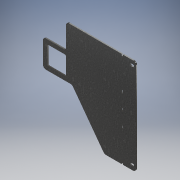
# Autodesk Inventor part: CAR SIDE PLATE II
Saved by Autodesk Inventor 2017 (Build 210142000, 142)
## iProperties
Part Number: CAR SIDE PLATE II
Material: Genérico
Document SubType Name: Modeling
Designer: Cristian
Density: 1 g/cm^3
Appearance: Valor por defecto
Author: Cristian
Autodesk Inventor part; units mm, degrees
ref_plane "YZ Plane" through (0, 0, 0) normal (1, 0, 0) x (0, 1, 0)
ref_plane "XZ Plane" through (0, 0, 0) normal (0, 1, 0) x (-1, 0, 0)
ref_plane "XY Plane" through (0, 0, 0) normal (0, 0, 1) x (1, 0, 0)
sketch "Boceto1" plane through (0, 0, 0) normal (0, 1, 0) x (-1, 0, 0)
  line L0 (0, 0) -> (288.925, 0)
  line L1 (288.925, 0) -> (288.925, -101.6)
  line L2 (288.925, -101.6) -> (384.175, -101.6)
  line L3 (384.175, -101.6) -> (384.175, -212.725)
  line L4 (0, 0) -> (0, -393.7)
  line L5 (0, -393.7) -> (130.175, -393.7)
  line L6 (384.175, -212.725) -> (263.525, -212.725)
  line L7 (263.525, -212.725) -> (130.175, -393.7)
  dimension "d0" = 288.925
  dimension "d1" = 101.6
  dimension "d2" = 95.25
  dimension "d3" = 111.125
  dimension "d4" = 393.7
  dimension "d50" = 130.175
  dimension "d51" = 133.35
  constraints: 16 end point, 3 horizontal, 2 perpendicular, 2 vertical
  measures "d0" distance of L0.start L0.end
  measures "d1" distance of L0.end L1.end
  measures "d2" distance of L1.end L2.end
  measures "d3" distance of L2.end L3.end
  measures "d4" distance of L0.start L4.end
  measures "d50" distance of L4.end L5.end
  measures "d51" horizontal distance of L5.end L6.end
extrude "Extrusión1" add sketch "Boceto1" along normal blind 5
fillet "Empalme1" radius 12.7 7 edges at (-384.175, 2.5, -101.6) (-288.925, 2.5, 0) (-384.175, 2.5, -212.725) (-263.525, 2.5, -212.725) (-130.175, 2.5, -393.7) (0, 2.5, -393.7) (0, 2.5, 0)
fillet "Empalme2" radius 6.35 1 edges at (-288.925, 2.5, -101.6)
sketch "Boceto2" plane through (0, 5, 0) normal (0, 1, 0) x (1, 0, 0)
  line L0 (-365.125, 119.0625) -> (-288.925, 119.0625)
  line L1 (-288.925, 119.0625) -> (-288.925, 195.2625)
  line L2 (-288.925, 195.2625) -> (-365.125, 195.2625)
  line L3 (-365.125, 195.2625) -> (-365.125, 119.0625)
  line L4 (-384.175, 200.025) -> (-384.175, 114.3) projected
  line L5 (-269.9424, 212.725) -> (-371.475, 212.725) projected
  line L6 (-371.475, 101.6) -> (-295.275, 101.6) projected
  line L7 (-276.225, 0) -> (-12.7, 0) projected
  line L8 (-59.5312, 0) -> (-53.975, 0)
  line L9 (-53.975, 0) -> (-53.975, 6.35)
  line L10 (-53.975, 6.35) -> (-59.5312, 6.35)
  line L11 (-59.5312, 6.35) -> (-59.5312, 0)
  line L12 (-12.7, 393.7) -> (-123.7576, 393.7) projected
  line L13 (0, 12.7) -> (0, 381) projected
  circle A0 centre (-15.875, 374.65) radius 5
  circle A1 centre (-15.875, 19.05) radius 5
  line L14 (-123.7576, 393.7) -> (-12.7, 393.7) projected
  line L15 (-59.5313, 393.7) -> (-53.975, 393.7)
  line L16 (-53.975, 393.7) -> (-53.975, 387.35)
  line L17 (-53.975, 387.35) -> (-59.5313, 387.35)
  line L18 (-59.5313, 387.35) -> (-59.5313, 393.7)
  line L19 (-59.5313, 127) -> (-53.975, 127)
  line L20 (-53.975, 127) -> (-53.975, 140.0969)
  line L21 (-53.975, 140.0969) -> (-59.5313, 140.0969)
  line L22 (-59.5313, 140.0969) -> (-59.5313, 127)
  line L23 (-59.5313, 190.5) -> (-53.975, 190.5)
  line L24 (-53.975, 190.5) -> (-53.975, 203.5969)
  line L25 (-53.975, 203.5969) -> (-59.5313, 203.5969)
  line L26 (-59.5313, 203.5969) -> (-59.5313, 190.5)
  line L27 (-59.5313, 254) -> (-53.975, 254)
  line L28 (-53.975, 254) -> (-53.975, 267.0969)
  line L29 (-53.975, 267.0969) -> (-59.5313, 267.0969)
  line L30 (-59.5313, 267.0969) -> (-59.5313, 254)
  circle A2 centre (-19.6062, 19.05) radius 5
  circle A3 centre (-12.1438, 19.05) radius 5
  line L31 (-19.6062, 19.05) -> (-15.875, 19.05)
  line L32 (-15.875, 19.05) -> (-12.1438, 19.05)
  line L33 (-19.6062, 14.05) -> (-12.1437, 14.05)
  line L34 (-19.6062, 24.05) -> (-12.1437, 24.05)
  circle A4 centre (-19.6063, 374.65) radius 5
  circle A5 centre (-12.1438, 374.65) radius 5
  line L35 (-19.6063, 374.65) -> (-15.875, 374.65)
  line L36 (-15.875, 374.65) -> (-12.1438, 374.65)
  line L37 (-19.6063, 369.65) -> (-12.1437, 369.65)
  line L38 (-19.6063, 379.65) -> (-12.1438, 379.65)
  point P0 (0, 0)
  dimension "d11" = 76.2
  dimension "d17" = 17.4625
  dimension "d18" = 19.05
  dimension "d19" = 76.2
  dimension "d20" = 5.5563
  dimension "d22" = 6.35
  dimension "d24" = 53.975
  dimension "d42" = 10
  dimension "d43" = 19.05
  dimension "d44" = 15.875
  dimension "d47" = 10
  dimension "d52" = 53.975
  dimension "d53" = 5.5563
  dimension "d54" = 6.35
  dimension "d67" = 15.875
  dimension "d68" = 19.05
  dimension "d69" = 5.5563
  dimension "d70" = 5.5563
  dimension "d71" = 5.5563
  dimension "d72" = 13.0969
  dimension "d73" = 13.0969
  dimension "d74" = 13.0969
  dimension "d75" = 53.975
  dimension "d80" = 63.5
  dimension "d81" = 63.5
  dimension "d82" = 127
  dimension "d87" = 10
  dimension "d88" = 10
  dimension "d89" = 17.4625
  dimension "d90" = 10
  dimension "d91" = 10
  dimension "d92" = 17.4625
  constraints: 64 end point, 15 equal length, 10 horizontal, 8 point on circle, 6 centre point, 6 perpendicular, 5 tangent, 3 collinear, 3 point on line
  measures "d11" distance of L2.end L0.start
  measures "d17" distance between parallel lines of L0 L6
  measures "d18" distance between parallel lines of L3 L4
  measures "d19" distance of L1.end L2.end
  measures "d20" distance between parallel lines of L9 L11
  measures "d22" distance of L10.end L8.start
  measures "d24" distance between parallel lines of L13 L9
  measures "d42" diameter of A0
  measures "d43" distance from line of L12 L35.end
  measures "d44" distance from line of L13 L35.end
  measures "d47" diameter of A1
  measures "d52" distance between parallel lines of L13 L16
  measures "d53" distance between parallel lines of L16 L18
  measures "d54" distance of L17.end L15.start
  measures "d67" distance from line of L13 L31.end
  measures "d68" distance from line of L7 L31.end
  measures "d69" distance of L21.end L20.end
  measures "d70" distance of L25.end L24.end
  measures "d71" distance between parallel lines of L28 L30
  measures "d72" distance between parallel lines of L21 L19
  measures "d73" distance of L23.end L24.end
  measures "d74" distance of L27.end L28.end
  measures "d75" distance between parallel lines of L13 L20
  measures "d80" distance between parallel lines of L23 L19
  measures "d81" distance between parallel lines of L27 L23
  measures "d82" distance between parallel lines of L7 L19
  measures "d87" diameter of A2
  measures "d88" diameter of A3
  measures "d90" diameter of A4
  measures "d91" diameter of A5
extrude "Extrusión2" cut sketch "Boceto2" against normal up to next
fillet "Empalme3" radius 3.5719 4 edges at (-365.125, 2.5, -119.0625) (-365.125, 2.5, -195.2625) (-288.925, 2.5, -195.2625) (-288.925, 2.5, -119.0625)
equation "\"d42\" = UBD"
equation "\"d47\" = UBD"
equation "\"d87\" = UBD"
equation "\"d88\" = UBD"
equation "\"d89\" = BTOL"
equation "\"d90\" = UBD"
equation "\"d91\" = UBD"
equation "\"d92\" = BTOL"
equation "\"LM\" = 76.2"
equation "\"UBD\" = 10"
equation "\"BTOL\" = 17.4625"
